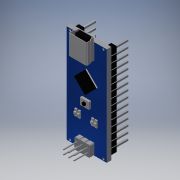
# Autodesk Inventor part: Arduino Nano
Saved by Autodesk Inventor 2017 (Build 210142000, 142)
## iProperties
Created: 2017-06-10
Part Number: Arduino Nano
Material: Generic
Document SubType Name: Modeling
Designer: L.Đ.P
Density: 1 g/cm^3
Appearance: Default
Author: L.Đ.P
Autodesk Inventor part; units mm, degrees
ref_plane "YZ Plane" through (0, 0, 0) normal (1, 0, 0) x (0, 1, 0)
ref_plane "XZ Plane" through (0, 0, 0) normal (0, 1, 0) x (-1, 0, 0)
ref_plane "XY Plane" through (0, 0, 0) normal (0, 0, 1) x (1, 0, 0)
sketch "Sketch1" plane through (0, 0, 0) normal (0, 1, 0) x (-1, 0, 0)
  line L0 (9, -22) -> (-9, -22)
  line L1 (-9, -22) -> (-9, 22)
  line L2 (-9, 22) -> (9, 22)
  line L3 (9, 22) -> (9, -22)
  line L4 (0, 0) -> (0, 11.2102)
  line L5 (0, 0) -> (7.3333, 0)
  point P0 (0, 22)
  point P1 (9, 0)
  dimension "d0" = 18
  dimension "d1" = 44
  constraints: 12 end point, 3 parallel, 2 midpoint, 2 perpendicular, 2 point on line, 1 horizontal
  measures "d0" distance of L1.end L2.end
  measures "d1" distance of L0.end L1.end
extrude "Extrusion1" add sketch "Sketch1" along normal blind 2
sketch "Sketch2" plane through (0, 2, 0) normal (0, 1, 0) x (1, 0, 0)
  line L0 (9, 22) -> (-9, 22) projected
  line L1 (-9, 22) -> (-9, -22) projected
  line L2 (-6, 18) -> (-8.5, 18)
  line L3 (-8.5, 18) -> (-8.5, 20.5)
  line L4 (-8.5, 20.5) -> (-6, 20.5)
  line L5 (-6, 20.5) -> (-6, 18)
  point P0 (0, 0)
  dimension "d4" = 2.5
  dimension "d5" = 2.5
  dimension "d6" = 1.5
  dimension "d7" = 0.5
  constraints: 8 end point, 2 parallel, 1 horizontal, 1 perpendicular
  measures "d4" distance of L3.end L4.end
  measures "d5" distance of L2.end L3.end
  measures "d6" distance between parallel lines of L0 L4
  measures "d7" distance between parallel lines of L1 L3
extrude "Extrusion2" add sketch "Sketch2" along normal blind 3
sketch "Sketch3" plane through (0, 5, 0) normal (0, 1, 0) x (1, 0, 0)
  line L0 (-6, 20.5) -> (-8.5, 20.5) projected
  line L1 (-8.5, 20.5) -> (-8.5, 18) projected
  line L2 (-6.875, 18.875) -> (-7.625, 18.875)
  line L3 (-7.625, 18.875) -> (-7.625, 19.625)
  line L4 (-7.625, 19.625) -> (-6.875, 19.625)
  line L5 (-6.875, 19.625) -> (-6.875, 18.875)
  line L6 (-7.25, 20.5) -> (-7.25, 19.7838)
  line L7 (-8.5, 19.25) -> (-8.011, 19.25)
  point P0 (0, 0)
  point P1 (-7.625, 19.25)
  point P2 (-7.25, 19.625)
  dimension "d10" = 0.75
  dimension "d11" = 0.75
  constraints: 12 end point, 4 midpoint, 3 parallel, 2 perpendicular, 2 point on line, 1 horizontal
  measures "d10" distance of L3.end L4.end
  measures "d11" distance of L2.end L3.end
extrude "Extrusion3" add sketch "Sketch3" along normal blind 6
pattern_linear "Rectangular Pattern1" count 15 spacing 2.75 along (0, 0, 1) of "Extrusion2", "Extrusion3"
mirror "Mirror1" about plane through (0, 0, 0) normal (1, 0, 0) of "Extrusion2", "Extrusion3", "Rectangular Pattern1"
sketch "Sketch4" plane through (0, 2, 0) normal (0, 1, 0) x (1, 0, 0)
  line L0 (9, 22) -> (-9, 22) projected
  line L1 (9, -22) -> (9, 22) projected
  circle A0 centre (7.5, 21.25) radius 0.5
  line L2 (0, 0) -> (0, 2.75)
  line L3 (0, 0) -> (3.2686, 0)
  circle A1 centre (-7.5, 21.25) radius 0.5
  circle A2 centre (7.5, -21.25) radius 0.5
  circle A3 centre (-7.5, -21.25) radius 0.5
  dimension "d17" = 1
  dimension "d18" = 1.5
  dimension "d19" = 0.75
  constraints: 4 centre point, 4 end point, 3 symmetric about line, 1 parallel, 1 perpendicular, 3 other
  measures "d17" diameter of A0
  measures "d18" distance from line of L1 A0.centre
  measures "d19" distance from line of L0 A0.centre
extrude "Extrusion4" cut sketch "Sketch4" against normal through all
sketch "Sketch5" plane through (0, 0, 0) normal (0, -1, 0) x (1, 0, 0)
  line L0 (-9, -22) -> (9, -22) projected
  line L1 (3.5, -22) -> (-3.5, -22)
  line L2 (-3.5, -22) -> (-3.5, -17)
  line L3 (-3.5, -17) -> (3.5, -17)
  line L4 (3.5, -17) -> (3.5, -22)
  line L5 (-3.5, -17.3536) -> (-3.1464, -17)
  line L6 (-1.5, -17) -> (-1.1464, -17.3536)
  line L7 (-1.1464, -17.3536) -> (-0.7929, -17)
  line L8 (0.7929, -17) -> (1.1464, -17.3536)
  line L9 (1.1464, -17.3536) -> (1.5, -17)
  line L10 (3.1464, -17) -> (3.5, -17.3536)
  line L11 (-3.5, -21.6464) -> (-3.1464, -22)
  line L12 (-1.5, -22) -> (-1.1464, -21.6464)
  line L13 (-1.1464, -21.6464) -> (-0.7929, -22)
  line L14 (0.7929, -22) -> (1.1464, -21.6464)
  line L15 (1.1464, -21.6464) -> (1.5, -22)
  line L16 (3.5, -21.6464) -> (3.1464, -22)
  point P0 (0, 0)
  point P1 (0, -22)
  dimension "d22" = 7
  dimension "d23" = 5
  dimension "d24" = 0.5
  dimension "d25" = 45
  dimension "d26" = 2
  dimension "d27" = 2
  dimension "d28" = 2
  dimension "d29" = 2
  constraints: 30 end point, 16 perpendicular, 10 point on line, 3 parallel, 1 horizontal, 1 midpoint, 1 vertical, 10 other
  measures "d22" distance of L2.end L3.end
  measures "d23" distance of L2.start L2.end
  measures "d24" distance of L5.start L5.end
  measures "d25" angle of L3 L5
  measures "d26" horizontal distance of L5.end L6.end
  measures "d27" horizontal distance of L8.end L10.start
  measures "d28" horizontal distance of L12.end L11.end
  measures "d29" horizontal distance of L16.end L14.end
extrude "Extrusion5" add sketch "Sketch5" along normal blind 2 contours L11 L2 L5 L3 L6 L7 L8 L9 L10 L4 L16 L0 L15 L14 L13 L12
sketch "Sketch6" plane through (0, -2, 0) normal (0, -1, 0) x (1, 0, 0)
  line L0 (3.1464, -17) -> (1.5, -17) projected
  line L1 (0.7929, -17) -> (-0.7929, -17) projected
  line L2 (-1.5, -17) -> (-3.1464, -17) projected
  line L3 (-3.5, -17.3536) -> (-3.5, -21.6464) projected
  line L4 (-3.1464, -22) -> (-1.5, -22) projected
  circle A0 centre (2.3232, -18.5) radius 0.25
  line L5 (2.3232, -17) -> (2.3232, -16.3121)
  line L6 (0, -17) -> (0, -16.3121)
  line L7 (-2.3232, -17) -> (-2.3232, -16.3121)
  circle A1 centre (0, -18.5) radius 0.25
  circle A2 centre (-2.3232, -18.5) radius 0.25
  line L8 (-3.5, -19.5) -> (-4.2081, -19.5)
  circle A3 centre (2.3232, -20.5) radius 0.25
  circle A4 centre (0, -20.5) radius 0.25
  circle A5 centre (-2.3232, -20.5) radius 0.25
  point P0 (0, 0)
  dimension "d32" = 0.5
  dimension "d34" = 1.5
  dimension "d35" = 0.5
  dimension "d36" = 0.5
  dimension "d37" = 1.5
  dimension "d38" = 1.5
  constraints: 8 end point, 6 centre point, 4 midpoint, 3 point on line, 3 symmetric about line, 2 parallel, 2 perpendicular, 3 other
  measures "d32" diameter of A0
  measures "d34" distance from line of L0 A0.centre
  measures "d35" diameter of A1
  measures "d36" diameter of A2
  measures "d37" distance from line of L1 A1.centre
  measures "d38" distance from line of L2 A2.centre
extrude "Extrusion6" add sketch "Sketch6" along normal blind 6
sketch "Sketch7" plane through (-9, 0, 22) normal (0, 0, 1) x (1, 0, 0)
  line L0 (18, 0) -> (0, 0) projected
  line L1 (5.5, 0) -> (12.5, 0)
  line L2 (12.5, 0) -> (12.5, -2)
  line L3 (12.5, -2) -> (5.5, -2)
  line L4 (5.5, -2) -> (5.5, 0)
  line L5 (5, -2) -> (13, -2)
  line L6 (13, -2) -> (13, -4)
  line L7 (13, -4) -> (5, -4)
  line L8 (5, -4) -> (5, -2)
  point P0 (9, 0)
  point P1 (9, -2)
  point P2 (9, 0)
  dimension "d41" = 7
  dimension "d42" = 2
  dimension "d43" = 8
  dimension "d44" = 2
  constraints: 16 end point, 4 midpoint, 4 parallel, 2 horizontal, 2 perpendicular
  measures "d41" distance of L2.end L3.end
  measures "d42" distance of L1.end L2.end
  measures "d43" distance of L6.end L7.end
  measures "d44" distance of L5.end L6.end
extrude "Extrusion7" add sketch "Sketch7" along normal blind 2 and the other way blind 7
fillet "Fillet1" radius 0.5 8 edges at (-3.5, -2, 19.5) (-4, -2, 19.5) (-4, -4, 19.5) (4, -4, 19.5) (4, -2, 19.5) (3.5, -2, 19.5) (-3.5, 0, 23) (3.5, 0, 23)
sketch "Sketch8" plane through (0, 0, 0) normal (0, -1, 0) x (1, 0, 0)
  line L0 (-3.5, 22) -> (-9, 22) projected
  line L1 (3.5, -21.6464) -> (3.1464, -22) projected
  line L2 (3.5, 15) -> (-3.5, 15) projected
  line L3 (0, 10) -> (-4.9497, 5.0503)
  line L4 (-4.9497, 5.0503) -> (0, 0.1005)
  line L5 (0, 0.1005) -> (4.9497, 5.0503)
  line L6 (4.9497, 5.0503) -> (0, 10)
  line L7 (0, 0) -> (0, -5.4813)
  dimension "d50" = 7
  dimension "d51" = 12
  constraints: 10 end point, 3 parallel, 3 perpendicular, 1 point on line
  measures "d50" distance of L3.end L4.end
  measures "d51" distance from line of L0 L3.start
extrude "Extrusion8" add sketch "Sketch8" along normal blind 1
fillet "Fillet2" radius 0.5 4 edges at (-2.4749, -1, 2.5754) (-2.4749, -1, 7.5251) (2.4749, -1, 7.5251) (2.4749, -1, 2.5754)
sketch "Sketch9" plane through (0, 0, 0) normal (0, -1, 0) x (1, 0, 0)
  line L0 (2, -4.5) -> (-2, -4.5)
  line L1 (-2, -4.5) -> (-2, -1.5)
  line L2 (-2, -1.5) -> (2, -1.5)
  line L3 (2, -1.5) -> (2, -4.5)
  line L4 (0, 10) -> (0, 6.7922)
  point P0 (0, 0)
  point P1 (0, -4.5)
  dimension "d55" = 4
  dimension "d56" = 3
  dimension "d58" = 1.5
  constraints: 10 end point, 3 parallel, 1 horizontal, 1 midpoint, 1 perpendicular, 1 point on line
  measures "d55" distance of L1.end L2.end
  measures "d56" distance of L0.end L1.end
  measures "d58" distance from line of L2 point (0, 0)
extrude "Extrusion9" add sketch "Sketch9" along normal blind 1
sketch "Sketch10" plane through (0, -1, 0) normal (0, -1, 0) x (1, 0, 0)
  line L0 (2, -1.5) -> (-2, -1.5) projected
  line L1 (-2, -1.5) -> (-2, -4.5) projected
  circle A0 centre (0, -3) radius 0.75
  line L2 (0, -1.5) -> (0, -1.0388)
  line L3 (-2, -3) -> (-2.4187, -3)
  point P0 (0, 0)
  dimension "d61" = 1.5
  constraints: 4 end point, 2 midpoint, 2 point on line, 1 centre point, 1 parallel, 1 perpendicular
  measures "d61" diameter of A0
extrude "Extrusion10" add sketch "Sketch10" along normal blind 0.5
sketch "Sketch11" plane through (0, 0, 0) normal (0, -1, 0) x (1, 0, 0)
  line L0 (2, -4.5) -> (-2, -4.5) projected
  line L1 (-9, 22) -> (-9, -22) projected
  line L2 (-4, -10.5) -> (-5, -10.5)
  line L3 (-5, -10.5) -> (-5, -7.5)
  line L4 (-5, -7.5) -> (-4, -7.5)
  line L5 (-4, -7.5) -> (-4, -10.5)
  line L6 (-2.5, -10.5) -> (-3.5, -10.5)
  line L7 (-3.5, -10.5) -> (-3.5, -7.5)
  line L8 (-3.5, -7.5) -> (-2.5, -7.5)
  line L9 (-2.5, -7.5) -> (-2.5, -10.5)
  line L10 (0, -4.5) -> (0, -6.1387)
  line L11 (-4, -9.5) -> (-5, -9.5)
  line L12 (-5, -9.5) -> (-5, -8.5)
  line L13 (-5, -8.5) -> (-4, -8.5)
  line L14 (-4, -8.5) -> (-4, -9.5)
  line L15 (-2.5, -9.5) -> (-3.5, -9.5)
  line L16 (-3.5, -9.5) -> (-3.5, -8.5)
  line L17 (-3.5, -8.5) -> (-2.5, -8.5)
  line L18 (-2.5, -8.5) -> (-2.5, -9.5)
  line L19 (4, -10.5) -> (5, -10.5)
  line L20 (5, -10.5) -> (5, -7.5)
  line L21 (5, -7.5) -> (4, -7.5)
  line L22 (4, -7.5) -> (4, -10.5)
  line L23 (2.5, -10.5) -> (3.5, -10.5)
  line L24 (3.5, -10.5) -> (3.5, -7.5)
  line L25 (3.5, -7.5) -> (2.5, -7.5)
  line L26 (2.5, -7.5) -> (2.5, -10.5)
  line L27 (4, -9.5) -> (5, -9.5)
  line L28 (5, -9.5) -> (5, -8.5)
  line L29 (5, -8.5) -> (4, -8.5)
  line L30 (4, -8.5) -> (4, -9.5)
  line L31 (2.5, -9.5) -> (3.5, -9.5)
  line L32 (3.5, -9.5) -> (3.5, -8.5)
  line L33 (3.5, -8.5) -> (2.5, -8.5)
  line L34 (2.5, -8.5) -> (2.5, -9.5)
  point P0 (0, 0)
  point P1 (-5, -9)
  point P2 (-4, -9)
  point P3 (-3.5, -9)
  point P4 (-2.5, -9)
  point P5 (5, -9)
  point P6 (4, -9)
  point P7 (3.5, -9)
  point P8 (2.5, -9)
  dimension "d64" = 1
  dimension "d65" = 3
  dimension "d66" = 3
  dimension "d67" = 4
  dimension "d68" = 1
  dimension "d69" = 3
  dimension "d70" = 0.5
  dimension "d71" = 1
  dimension "d72" = 1
  constraints: 66 end point, 20 symmetric about line, 9 midpoint, 9 parallel, 4 horizontal, 4 perpendicular, 1 collinear
  measures "d64" distance of L3.end L4.end
  measures "d65" distance of L2.end L3.end
  measures "d66" distance between parallel lines of L4 L0
  measures "d67" distance between parallel lines of L1 L3
  measures "d68" distance of L7.end L8.end
  measures "d69" distance of L6.end L7.end
  measures "d70" distance between parallel lines of L7 L5
  measures "d71" distance of L11.end L12.end
  measures "d72" distance of L15.end L16.end
extrude "Extrusion11" add sketch "Sketch11" along normal blind 0.5
extrude "Extrusion12" add sketch "Sketch11" along normal blind 1 contours L11 L3 L13 L5 | L15 L7 L17 L9 | L22 L29 L20 L27 | L26 L33 L24 L31
sketch "Sketch13" plane through (0, 2, 0) normal (0, 1, 0) x (1, 0, 0)
  line L0 (-9, -22) -> (9, -22) projected
  line L1 (9, -22) -> (9, 22) projected
  line L2 (3, -19) -> (4, -19)
  line L3 (4, -19) -> (4, -21)
  line L4 (4, -21) -> (3, -21)
  line L5 (3, -21) -> (3, -19)
  line L6 (-1.5, -20.8812) -> (1.5, -20.8812)
  line L7 (1.5, -20.8812) -> (1.5, -21.8812)
  line L8 (1.5, -21.8812) -> (-1.5, -21.8812)
  line L9 (-1.5, -21.8812) -> (-1.5, -20.8812)
  line L10 (-2.5462, -21) -> (-3.5462, -21)
  line L11 (-3.5462, -21) -> (-3.5462, -19)
  line L12 (-3.5462, -19) -> (-2.5462, -19)
  line L13 (-2.5462, -19) -> (-2.5462, -21)
  line L14 (-4.9079, -19) -> (-3.9079, -19)
  line L15 (-3.9079, -19) -> (-3.9079, -21)
  line L16 (-3.9079, -21) -> (-4.9079, -21)
  line L17 (-4.9079, -21) -> (-4.9079, -19)
  point P0 (0, 0)
  dimension "d77" = 1
  dimension "d78" = 2
  dimension "d79" = 3
  dimension "d80" = 1
  dimension "d81" = 1
  dimension "d82" = 2
  dimension "d83" = 1
  dimension "d84" = 2
  dimension "d85" = 1
  dimension "d86" = 5
  constraints: 32 end point, 8 parallel, 4 horizontal, 4 perpendicular, 2 collinear
  measures "d77" distance of L3.end L4.end
  measures "d78" distance of L2.end L3.end
  measures "d79" distance of L7.end L8.end
  measures "d80" distance of L6.end L7.end
  measures "d81" distance of L11.end L12.end
  measures "d82" distance of L10.end L11.end
  measures "d83" distance of L15.end L16.end
  measures "d84" distance of L14.end L15.end
  measures "d85" distance between parallel lines of L0 L4
  measures "d86" distance between parallel lines of L1 L3
extrude "Extrusion13" add sketch "Sketch13" along normal blind 0.5
sketch "Sketch14" plane through (0, 2, 0) normal (0, 1, 0) x (1, 0, 0)
  line L0 (1.5, -22) -> (9, -22) projected
  line L1 (9, -22) -> (9, 22) projected
  line L2 (4, -17.5) -> (0, -17.5)
  line L3 (0, -17.5) -> (0, -7.5)
  line L4 (0, -7.5) -> (4, -7.5)
  line L5 (4, -7.5) -> (4, -17.5)
  point P0 (1.5, -21.8812)
  point P1 (0, 0)
  dimension "d89" = 4
  dimension "d90" = 10
  dimension "d91" = 4.5
  dimension "d92" = 5
  constraints: 8 end point, 2 parallel, 1 horizontal, 1 perpendicular
  measures "d89" distance of L3.end L4.end
  measures "d90" distance of L2.end L3.end
  measures "d91" distance between parallel lines of L0 L2
  measures "d92" distance between parallel lines of L1 L5
extrude "Extrusion14" add sketch "Sketch14" along normal blind 0.5
sketch "Sketch15" plane through (0, 2, 0) normal (0, 1, 0) x (1, 0, 0)
  line L0 (9, 22) -> (-9, 22) projected
  line L1 (2.5, 16) -> (-2.5, 16)
  line L2 (-2.5, 16) -> (-2.5, 13)
  line L3 (-2.5, 13) -> (2.5, 13)
  line L4 (2.5, 13) -> (2.5, 16)
  line L5 (0, 0) -> (0, 2.2721)
  point P0 (0, 13)
  dimension "d95" = 5
  dimension "d96" = 3
  dimension "d97" = 6
  constraints: 10 end point, 3 parallel, 1 horizontal, 1 midpoint, 1 perpendicular, 1 point on line
  measures "d95" distance of L3.end L2.end
  measures "d96" distance of L2.end L1.end
  measures "d97" distance between parallel lines of L0 L1
extrude "Extrusion15" add sketch "Sketch15" along normal blind 0.5
sketch "Sketch16" plane through (-9, 0, 24) normal (0, 0, 1) x (1, 0, 0)
  arc A0 (13, -2.366) -> (12.75, -1.933) centre (12.5, -2.366) ccw projected
  arc A1 (12.5, -1.5) -> (12.75, -1.933) centre (13, -1.5) ccw projected
  line L0 (12.5, -1.5) -> (12.5, -0.5) projected
  arc A2 (12.5, -0.5) -> (12, 0) centre (12, -0.5) ccw projected
  line L1 (12, 0) -> (6, 0) projected
  arc A3 (6, 0) -> (5.5, -0.5) centre (6, -0.5) ccw projected
  line L2 (5.5, -0.5) -> (5.5, -1.5) projected
  arc A4 (5.25, -1.933) -> (5.5, -1.5) centre (5, -1.5) ccw projected
  arc A5 (5.25, -1.933) -> (5, -2.366) centre (5.5, -2.366) ccw projected
  line L3 (5, -2.366) -> (5, -3.5) projected
  arc A6 (5, -3.5) -> (5.5, -4) centre (5.5, -3.5) ccw projected
  line L4 (5.5, -4) -> (12.5, -4) projected
  arc A7 (12.5, -4) -> (13, -3.5) centre (12.5, -3.5) ccw projected
  line L5 (13, -3.5) -> (13, -2.366) projected
  line L6 (11.5, -2.5) -> (6.5, -2.5)
  line L7 (6.5, -2.5) -> (6.5, -0.5)
  line L8 (6.5, -0.5) -> (11.5, -0.5)
  line L9 (11.5, -0.5) -> (11.5, -2.5)
  line L10 (9, 0) -> (9, 1.8012)
  line L11 (6, -0.2) -> (12, -0.2)
  arc A8 (12.3, -0.5) -> (12, -0.2) centre (12, -0.5) ccw
  line L12 (12.3, -0.5) -> (12.3, -1.5)
  arc A9 (12.3, -1.5) -> (12.65, -2.1062) centre (13, -1.5) ccw
  arc A10 (12.8, -2.366) -> (12.65, -2.1062) centre (12.5, -2.366) ccw
  line L13 (12.8, -2.366) -> (12.8, -3.5)
  arc A11 (12.5, -3.8) -> (12.8, -3.5) centre (12.5, -3.5) ccw
  line L14 (12.5, -3.8) -> (5.5, -3.8)
  arc A12 (5.2, -3.5) -> (5.5, -3.8) centre (5.5, -3.5) ccw
  line L15 (5.2, -3.5) -> (5.2, -2.366)
  arc A13 (5.35, -2.1062) -> (5.2, -2.366) centre (5.5, -2.366) ccw
  arc A14 (5.35, -2.1062) -> (5.7, -1.5) centre (5, -1.5) ccw
  line L16 (5.7, -1.5) -> (5.7, -0.5)
  arc A15 (6, -0.2) -> (5.7, -0.5) centre (6, -0.5) ccw
  point P0 (9, -0.5)
  dimension "d100" = 5
  dimension "d101" = 2
  dimension "d102" = 0.5
  dimension "d103" = 0.2
  constraints: 22 end point, 16 point on circle, 8 centre point, 3 parallel, 1 horizontal, 1 midpoint, 1 perpendicular, 1 point on line, 13 other
  measures "d100" distance of L7.end L8.end
  measures "d101" distance of L6.end L7.end
  measures "d102" distance between parallel lines of L1 L8
  measures "d103" distance between parallel lines of L1 L11
extrude "Extrusion16" cut sketch "Sketch16" against normal blind 8 contours L11 A8 L12 A9 A10 L13 A11 L14 A12 L15 A13 A14 L16 A15
body "Solid1"
